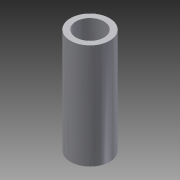
# Autodesk Inventor part: 凸轮套筒
Saved by Autodesk Inventor 2013 (Build 170138000, 138)
## iProperties
Created: 2012-10-03
Part Number: 凸轮套筒
Material: PVC 管
Document SubType Name: Modeling
Designer: Zhensheng
Density: 7.85 g/cm^3
Author: Zhensheng
Autodesk Inventor part; units mm, degrees
ref_plane "YZ Plane" through (0, 0, 0) normal (1, 0, 0) x (0, 1, 0)
ref_plane "XZ Plane" through (0, 0, 0) normal (0, 1, 0) x (-1, 0, 0)
ref_plane "XY Plane" through (0, 0, 0) normal (0, 0, 1) x (1, 0, 0)
sketch "草图1" plane through (0, 0, 0) normal (0, 0, 1) x (1, 0, 0)
  circle A0 centre (0, 0) radius 5
  circle A1 centre (0, 0) radius 7
  dimension "轴径" = 10
  dimension "外径" = 14
  constraints: 2 centre point, 2 coincident
  measures "轴径" diameter of A0
  measures "外径" diameter of A1
extrude "拉伸1" add sketch "草图1" along normal blind 37.5
